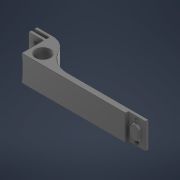
# Autodesk Inventor part: sensorbar
Saved by Autodesk Inventor 2022 (Build 260153000, 153)
## iProperties
Created: 2021-10-11
Part Number: sensorbar
Material: ABS プラスチック
Document SubType Name: Modeling
Designer: shiok
Density: 1.06 g/cm^3
Appearance: 滑らか - 白
Mass: 4.64134 g
Surface Area: 39.738 cm^2
Volume: 4.37862 cm^3
Author: shiok
Autodesk Inventor part; units mm, degrees
ref_plane "YZ Plane" through (0, 0, 0) normal (1, 0, 0) x (0, 1, 0)
ref_plane "XZ Plane" through (0, 0, 0) normal (0, 1, 0) x (-1, 0, 0)
ref_plane "XY Plane" through (0, 0, 0) normal (0, 0, 1) x (1, 0, 0)
sketch "スケッチ14" plane through (0, 0, 0) normal (0, 1, 0) x (-1, 0, 0)
  line L0 (0, -17.5) -> (-9.2265, -17.5)
  line L1 (-79, -3.2) -> (-79, 0)
  line L2 (-79, 0) -> (-9, 0)
  line L3 (0, -15.9) -> (-9, -15.9)
  line L4 (-17.8868, -12.5) -> (-18.926, -10.7)
  line L5 (-31.9164, -3.2) -> (-79, -3.2)
  line L6 (0, -15.9) -> (0, -17.5)
  line L7 (-9, -15.9) -> (-9, 0)
  arc A0 (-17.8868, -12.5) -> (-9.2265, -17.5) centre (-9.2265, -7.5) ccw
  arc A1 (-18.926, -10.7) -> (-31.9164, -3.2) centre (-31.9164, -18.2) ccw
  circle A2 centre (-14.9402, -5.9402) radius 4.3402
  line L8 (-14.9402, -1.6) -> (-14.9402, 0)
  line L9 (-10.6, -5.9402) -> (-9, -5.9402)
  line L10 (-18.4588, -8.4813) -> (-19.7559, -9.418)
  point P0 (0, 0)
  point P1 (-23.2561, -3.2)
  point P2 (-15, -17.5)
  dimension "d97" = 1.6
  dimension "d99" = 3.2
  dimension "d101" = 15
  dimension "d102" = 70
  dimension "d106" = 15.9
  dimension "d119" = 9
  dimension "d129" = 1.6
  dimension "d146" = 15
  dimension "d147" = 10
  dimension "d148" = 120
  constraints: 22 end point, 12 point on line, 8 point on circle, 5 perpendicular, 4 tangent, 3 centre point, 2 equal length, 2 horizontal, 2 parallel
  measures "d97" distance between parallel lines of L0 L3
  measures "d99" distance between parallel lines of L5 L2
  measures "d101" distance of point (-15, -17.5) L0.start
  measures "d102" distance of L2.end L1.end
  measures "d106" distance between parallel lines of L3 L2
  measures "d119" distance of L3.start L3.end
  measures "d129" distance of L9.start L9.end
  measures "d146" radius of A1
  measures "d147" radius of A0
  measures "d148" angle of L4 L5
extrude "押し出し5" add sketch "スケッチ14" along normal blind 15 contours L0 A0 L4 A1 L10 A2 L9 L7 L3 L6 | L9 A2 L8 L2 L7 | A1 L5 L1 L2 L8 A2 L10
sketch "スケッチ20" plane through (0, 0, 0) normal (0, -1, 0) x (1, 0, 0)
  line L0 (9, -15.9) -> (9, 0) projected
  line L1 (0, -15.9) -> (9, -15.9) projected
  line L2 (0, -17.5) -> (0, -15.9) projected
  line L3 (9.2265, -17.5) -> (0, -17.5) projected
  line L4 (18.926, -10.7) -> (17.8868, -12.5) projected
  line L5 (79, -3.2) -> (31.9164, -3.2) projected
  line L6 (79, 0) -> (79, -3.2) projected
  line L7 (9, 0) -> (79, 0) projected
  line L8 (9, -15.9) -> (9, 0) projected
  line L9 (0, -17.5) -> (0, -15.9) projected
  line L10 (11, -14.3) -> (0, -14.3)
  line L11 (0, -14.3) -> (0, -12.7)
  line L12 (0, -12.7) -> (11, -12.7)
  line L13 (11, -12.7) -> (11, -14.3)
  arc A0 (9.2265, -17.5) -> (17.8868, -12.5) centre (9.2265, -7.5) ccw projected
  arc A1 (31.9164, -3.2) -> (18.926, -10.7) centre (31.9164, -18.2) ccw projected
  point P0 (0, 0)
  dimension "d123" = 1.6
  dimension "d124" = 2
  constraints: 8 end point, 2 collinear, 2 parallel, 1 horizontal, 1 perpendicular
  measures "d123" distance between parallel lines of L1 L10
  measures "d124" distance between parallel lines of L0 L13
extrude "押し出し9" add sketch "スケッチ20" against normal up to surface (15 mm away) contours L10 L11 L12 L0 | L0 L12 L13 L10
sketch "スケッチ23" plane through (79, 0, 0) normal (0, 0, 1) x (1, 0, 0)
  line L0 (-70, 15) -> (0, 15) projected
  line L1 (0, 0) -> (-47.0836, 0) projected
  line L2 (0, 0) -> (-10, 0)
  line L3 (-10, 0) -> (-10, 15)
  line L4 (-10, 15) -> (0, 15)
  line L5 (0, 15) -> (0, 0)
  line L6 (-5.5, 11.25) -> (-5, 11.25)
  line L7 (-5, 11.25) -> (-5, 7.5) construction
  line L8 (-5, 7.5) -> (-7.5, 7.5) construction
  line L9 (-7.5, 7.5) -> (-7.5, 9.25)
  line L10 (-4.5, 11.25) -> (-5, 11.25)
  line L11 (-2.5, 7.5) -> (-2.5, 9.25)
  line L12 (-5.5, 3.75) -> (-5, 3.75)
  line L13 (-7.5, 7.5) -> (-7.5, 5.75)
  line L14 (-2.5, 7.5) -> (-2.5, 5.75)
  line L15 (-4.5, 3.75) -> (-5, 3.75)
  line L16 (-7.5, 7.5) -> (-10, 7.5) construction
  line L17 (-5, 11.25) -> (-5, 15) construction
  arc A0 (-5.5, 11.25) -> (-7.5, 9.25) centre (-5.5, 9.25) ccw
  arc A1 (-7.5, 5.75) -> (-5.5, 3.75) centre (-5.5, 5.75) ccw
  arc A2 (-4.5, 3.75) -> (-2.5, 5.75) centre (-4.5, 5.75) ccw
  arc A3 (-2.5, 9.25) -> (-4.5, 11.25) centre (-4.5, 9.25) ccw
  point P0 (-79, 0)
  point P1 (-7.5, 11.25)
  point P2 (-2.5, 11.25)
  point P3 (-7.5, 3.75)
  point P4 (-2.5, 3.75)
  dimension "d150" = 10
  dimension "d151" = 15
  dimension "d154" = 2
  constraints: 32 end point, 8 point on circle, 8 point on line, 8 tangent, 5 symmetric about line, 4 centre point, 4 collinear, 4 parallel, 3 equal radius, 2 horizontal, 2 midpoint, 2 perpendicular
  measures "d150" distance of L3.end L4.end
  measures "d151" distance of L2.end L3.end
  measures "d154" radius of A0
extrude "押し出し10" cut sketch "スケッチ23" against normal blind 1.6
sketch "スケッチ24" plane through (79, 0, -1.6) normal (0, 0, 1) x (1, 0, 0)
  line L0 (-10, 15) -> (0, 15) projected
  line L1 (-10, 0) -> (-10, 15) projected
  line L2 (0, 0) -> (-10, 0) projected
  line L3 (0, 15) -> (0, 0) projected
  line L4 (-7.5, 9.25) -> (-7.5, 5.75) projected
  arc A0 (-5.5, 11.25) -> (-7.5, 9.25) centre (-5.5, 9.25) ccw projected
  line L5 (-4.5, 11.25) -> (-5.5, 11.25) projected
  arc A1 (-2.5, 9.25) -> (-4.5, 11.25) centre (-4.5, 9.25) ccw projected
  line L6 (-2.5, 5.75) -> (-2.5, 9.25) projected
  arc A2 (-4.5, 3.75) -> (-2.5, 5.75) centre (-4.5, 5.75) ccw projected
  line L7 (-5.5, 3.75) -> (-4.5, 3.75) projected
  arc A3 (-7.5, 5.75) -> (-5.5, 3.75) centre (-5.5, 5.75) ccw projected
  arc A4 (-5.5, 11.25) -> (-7.5, 9.25) centre (-5.5, 9.25) ccw projected
  line L8 (-7.5, 9.25) -> (-7.5, 5.75) projected
  arc A5 (-7.5, 5.75) -> (-5.5, 3.75) centre (-5.5, 5.75) ccw projected
  line L9 (-5.5, 3.75) -> (-4.5, 3.75) projected
  arc A6 (-4.5, 3.75) -> (-2.5, 5.75) centre (-4.5, 5.75) ccw projected
  line L10 (-2.5, 5.75) -> (-2.5, 9.25) projected
  arc A7 (-2.5, 9.25) -> (-4.5, 11.25) centre (-4.5, 9.25) ccw projected
  line L11 (-4.5, 11.25) -> (-5.5, 11.25) projected
  line L12 (-5, 13.125) -> (-5, 15) construction
  line L13 (0, 15) -> (-47.0836, 15) construction
  line L14 (-5, 13.125) -> (-5, 11.25) construction
  line L15 (-4.5, 11.25) -> (-5.5, 11.25) construction
  line L16 (-5.5, 3.75) -> (-4.5, 3.75) construction
  line L17 (-5, 3.75) -> (-5, 1.875) construction
  line L18 (-5, 1.875) -> (-5, 0) construction
  line L19 (0, 0) -> (-47.0836, 0) construction
  point P0 (-79, 0)
  constraints: 8 end point, 5 collinear, 2 midpoint, 2 point on line, 1 perpendicular
hole "穴9" at (74, 1.875, -1.6) at (74, 13.125, -1.6) direction (0, 0, -1) diameter 2.013 depth 1.6 tip angle 118 thread size "M2.5x0.45" class "6H" standard "ISO Metric profile"
sketch "スケッチ25" plane through (9, 0, 0) normal (0, 0, 1) x (1, 0, 0)
  line L0 (0, 0) -> (0, 15) projected
  line L1 (60, 0) -> (60, 15) projected
  arc A0 (-0.4516, 0) -> (-0.4516, 15) centre (-62.5, 7.5) ccw
  line L2 (0, 0) -> (60, 0) projected
  line L3 (0, 15) -> (60, 15) projected
  line L4 (-0.4516, 15) -> (0, 15)
  line L5 (-0.4516, 0) -> (0, 0)
  line L6 (0, 0) -> (0, 15) projected
  line L7 (0, 7.5) -> (-62.5, 7.5)
  point P0 (0, 7.5)
  dimension "d166" = 62.5
  constraints: 6 end point, 2 horizontal, 2 point on circle, 2 point on line, 1 centre point, 1 coincident, 1 midpoint, 1 tangent
  measures "d166" distance of L7.start L7.end
extrude "押し出し11" add sketch "スケッチ25" against normal up to surface contours L5 A0 L0 | A0 L4 L0 round surface about axis through (9.2265, 0, -7.5) along (0, 1, 0) radius 10 far side no
sketch "スケッチ26" plane through (9.2265, 0, -17.5) normal (0, 0, -1) x (-1, 0, 0)
  line L0 (0, 0) -> (9.2265, 0) projected
  line L1 (9.2265, 0) -> (9.2265, 15) projected
  line L2 (0, 15) -> (9.2265, 15) projected
  line L3 (0, 0) -> (0, 15) projected
  line L4 (0, 0) -> (0, 15) projected
  line L5 (0, 7.5) -> (9.2265, 7.5)
  line L6 (9.2265, 0) -> (9.2265, 15) projected
  point P0 (5.2265, 3.75)
  point P1 (5.2265, 11.25)
  dimension "d169" = 4
  dimension "d170" = 3.75
  constraints: 2 end point, 2 midpoint, 1 symmetric about line
  measures "d169" distance from line of L1 point (5.226, 3.75)
  measures "d170" distance from line of L0 point (5.226, 3.75)
hole "穴10" at (4, 11.25, -17.5) at (4, 3.75, -17.5) direction (0, 0, 1) diameter 2.9 depth 1.6 tip angle 118 clearance for "Countersunk Flat Head Screw ISO 2009/7046" size "M2.5" standard "ISO"
sketch "スケッチ27" plane through (0, 0, -14.3) normal (0, 0, -1) x (-1, 0, 0)
  circle A0 centre (-4, 11.25) radius 1.5115 projected
  circle A1 centre (-4, 11.25) radius 0.889 projected
  circle A2 centre (-4, 3.75) radius 1.45 projected
  circle A3 centre (-4, 11.25) radius 1.45 projected
  point P0 (-4, 3.75)
  constraints: 2 coincident
hole "穴11" at (4, 11.25, -14.3) at (4, 3.75, -14.3) direction (0, 0, 1) diameter 2.1129 depth 1.6 tip angle 118 thread size "M2.6x0.45" class "6H" standard "ISO Metric profile"
